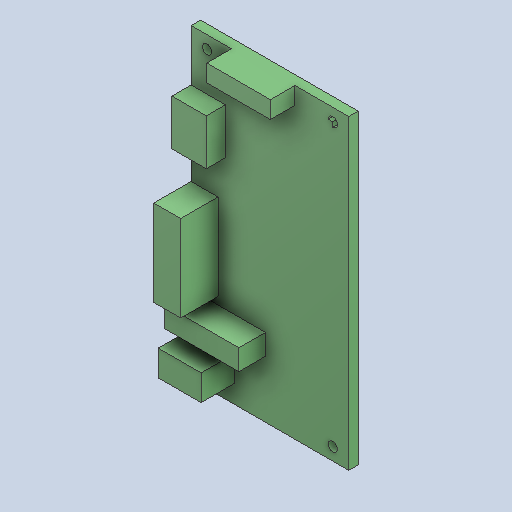
# Autodesk Inventor part: placa
Saved by Autodesk Inventor 2023 (Build 270158000, 158)
## iProperties
Created: 2023-05-12
Part Number: placa
Material: Genérico
Document SubType Name: Modeling
Designer: sergi
Density: 1 g/cm^3
Appearance: Valor por defecto
Author: sergi
Autodesk Inventor part; units mm, degrees
ref_plane "YZ Plane" through (0, 0, 0) normal (1, 0, 0) x (0, 1, 0)
ref_plane "XZ Plane" through (0, 0, 0) normal (0, 1, 0) x (-1, 0, 0)
ref_plane "XY Plane" through (0, 0, 0) normal (0, 0, 1) x (1, 0, 0)
sketch "Boceto1" plane through (0, 0, 0) normal (0, 0, 1) x (1, 0, 0)
  line L0 (27.55, -53.55) -> (-27.55, -53.55)
  line L1 (-27.55, -53.55) -> (-27.55, 53.55)
  line L2 (-27.55, 53.55) -> (27.55, 53.55)
  line L3 (27.55, 53.55) -> (27.55, -53.55)
  line L4 (27.55, -53.55) -> (-27.55, 53.55) construction
  line L5 (-27.55, -53.55) -> (27.55, 53.55) construction
  line L6 (20.325, -47.5) -> (-20.325, -47.5)
  line L7 (-20.325, -47.5) -> (-20.325, 47.5)
  line L8 (-20.325, 47.5) -> (20.325, 47.5)
  line L9 (20.325, 47.5) -> (20.325, -47.5)
  line L10 (20.325, -47.5) -> (-20.325, 47.5) construction
  line L11 (-20.325, -47.5) -> (20.325, 47.5) construction
  line L12 (-20.325, 47.5) -> (-21.975, 47.5)
  line L13 (-21.975, 47.5) -> (-21.975, 49.15)
  line L14 (-21.975, 49.15) -> (-21.975, -49.15)
  line L15 (-21.975, -49.15) -> (21.975, -49.15)
  line L16 (21.975, -49.15) -> (21.975, 49.15)
  line L17 (21.975, 49.15) -> (-21.975, 49.15)
  circle A0 centre (-21.975, 49.15) radius 1.65
  circle A1 centre (21.975, 49.15) radius 1.65
  circle A2 centre (21.975, -49.15) radius 1.65
  circle A3 centre (-21.975, -49.15) radius 1.65
  point P0 (0, 0)
  point P1 (20.325, 49.15)
  point P2 (21.975, 47.5)
  dimension "d0" = 55.1
  dimension "d1" = 107.1
  dimension "d2" = 40.65
  dimension "d3" = 95
  dimension "d4" = 1.65
  dimension "d5" = 1.65
  dimension "d6" = 1.65
  dimension "d7" = 3.3
  dimension "d8" = 3.3
  dimension "d9" = 3.3
  constraints: 36 end point, 6 parallel, 4 coincident, 4 midpoint, 4 perpendicular, 3 centre point, 3 horizontal, 1 vertical alignment, 5 other
  measures "d0" distance of L1.end L2.end
  measures "d1" distance of L0.end L1.end
  measures "d2" distance of L7.end L8.end
  measures "d3" distance of L6.end L7.end
  measures "d4" distance of L7.end L12.end
  measures "d5" distance of L12.end L13.end
  measures "d6" distance between parallel lines of L7 L14
  measures "d7" diameter of A1
  measures "d8" diameter of A2
  measures "d9" diameter of A3
extrude "Extrusión1" add sketch "Boceto1" along normal blind 16.35 contours L0 L1 L2 L3 | A0 L17 A1 L16 A2 L15 A3 L14 | L6 L7 L8 L9 | L17 L16 A1 picked at (20.8888, 49.0276)
sketch "Boceto2" plane through (-27.55, -53.55, 0) normal (-1, 0, 0) x (0, 0, 1)
  line L0 (0, 107.1) -> (0, 88.8)
  line L1 (0, 107.1) -> (0, 0) projected
  line L2 (0, 107.1) -> (3.3, 107.1)
  line L3 (3.3, 107.1) -> (3.3, 53.55)
  line L4 (3.3, 53.55) -> (3.3, 0)
  line L5 (0, 0) -> (16.35, 0) projected
  line L6 (3.3, 107.1) -> (11.9, 107.1)
  line L7 (0, 107.1) -> (16.35, 107.1) projected
  line L8 (11.9, 107.1) -> (11.9, 101.1)
  line L9 (11.9, 101.1) -> (3.3, 101.1)
  line L10 (3.3, 107.1) -> (3.3, 89.1)
  line L11 (0, 102.7) -> (16.35, 102.7) projected
  line L12 (3.3, 107.1) -> (21.3, 107.1) construction
  line L13 (3.3, 89.1) -> (10, 89.1)
  line L14 (10, 89.1) -> (10, 73.1)
  line L15 (10, 73.1) -> (3.3, 73.1)
  line L16 (3.3, 107.1) -> (3.3, 59.9)
  line L17 (3.3, 59.9) -> (16.3, 59.9)
  line L18 (16.3, 59.9) -> (16.35, 59.9)
  line L19 (16.35, 107.1) -> (16.35, 0) projected
  line L20 (16.35, 59.9) -> (16.35, 29.8)
  line L21 (16.35, 59.9) -> (46.45, 59.9) construction
  line L22 (16.35, 29.8) -> (3.3, 29.8)
  line L23 (3.3, 0) -> (3.3, 6.2)
  line L24 (3.3, 6.2) -> (14.8, 6.2)
  line L25 (16.35, 6.05) -> (0, 6.05) projected
  line L26 (3.3, 6.2) -> (14.8, 6.2) construction
  line L27 (14.8, 6.2) -> (14.8, 15.2)
  line L28 (14.8, 6.2) -> (23.8, 6.2) construction
  line L29 (14.8, 15.2) -> (3.3, 15.2)
  line L30 (3.3, 0) -> (3.3, 20)
  line L31 (3.3, 0) -> (23.3, 0) construction
  line L32 (3.3, 20) -> (12.6, 20)
  line L33 (12.6, 20) -> (12.6, 27.2)
  line L34 (12.6, 27.2) -> (3.3, 27.2)
  point P0 (0, 53.55)
  dimension "d17" = 3.3
  dimension "d18" = 8.6
  dimension "d19" = 6
  dimension "d20" = 18
  dimension "d21" = 90
  dimension "d22" = 6.7
  dimension "d23" = 16
  dimension "d24" = 47.2
  dimension "d25" = 13
  dimension "d26" = 90
  dimension "d27" = 30.1
  dimension "d28" = 90
  dimension "d29" = 6.2
  dimension "d30" = 11.5
  dimension "d31" = 0
  dimension "d32" = 9
  dimension "d33" = 90
  dimension "d34" = 20
  dimension "d35" = 90
  dimension "d36" = 9.3
  dimension "d37" = 90
  dimension "d38" = 7.2
  dimension "d39" = 90
  constraints: 58 end point, 13 point on line, 11 perpendicular, 5 equal length, 5 horizontal, 2 collinear, 2 vertical, 1 parallel
  measures "d17" distance of L0.start L2.end
  measures "d18" distance of L2.end L6.end
  measures "d19" distance of L6.end L8.end
  measures "d20" distance of L2.end L10.end
  measures "d21" angle of L10 L12
  measures "d22" distance of L10.end L13.end
  measures "d23" distance of L13.end L14.end
  measures "d24" distance of L2.end L16.end
  measures "d25" distance of L16.end L17.end
  measures "d26" angle of L17 L16
  measures "d27" distance of L18.end L20.end
  measures "d28" angle of L20 L21
  measures "d29" distance of L4.end L23.end
  measures "d30" distance of L23.end L24.end
  measures "d31" distance between parallel lines of L24 L26
  measures "d32" distance of L26.end L27.end
  measures "d33" angle of L28 L27
  measures "d34" distance of L4.end L30.end
  measures "d35" angle of L31 L30
  measures "d36" distance of L30.end L32.end
  measures "d37" angle of L30 L32
  measures "d38" distance of L32.end L33.end
  measures "d39" angle of L33 L32
extrude "Extrusión2" cut sketch "Boceto2" against normal through all contours L7 L19 L11 L8 | L9 L8 L11 L19 L18 L17 L3 L15 L14 L13 | L25 L19 L5 L4 | L4 L24 L27 L29 L32 L33 L34 L22 L19 L25
sketch "Boceto3" plane through (0, 0, 16.35) normal (0, 0, 1) x (1, 0, 0)
  line L0 (-27.55, 53.55) -> (27.55, 53.55) projected
  line L1 (27.55, 47.55) -> (27.55, 35.55) projected
  line L2 (27.55, 53.55) -> (27.55, 47.55) projected
  line L3 (27.55, 35.55) -> (27.55, 19.55) projected
  line L4 (27.55, 19.55) -> (27.55, 6.35) projected
  line L5 (27.55, -23.75) -> (27.55, 6.35) projected
  line L6 (27.55, -26.35) -> (27.55, -33.55) projected
  line L7 (-27.55, 53.55) -> (-27.55, -53.55) projected
  line L8 (27.55, 53.55) -> (-27.55, 53.55) projected
  line L9 (-27.55, -53.55) -> (27.55, -53.55) projected
  line L10 (27.55, -53.55) -> (27.55, 53.55) projected
  line L11 (-27.55, 53.55) -> (-13.45, 53.55)
  line L12 (-21.5719, 47.55) -> (21.975, 47.55) projected
  line L13 (-27.55, 35.55) -> (27.55, 35.55) projected
  line L14 (-27.55, 19.55) -> (27.55, 19.55) projected
  line L15 (-27.55, 6.35) -> (27.55, 6.35) projected
  line L16 (-27.55, -23.75) -> (27.55, -23.75) projected
  line L17 (-27.55, -26.35) -> (27.55, -26.35) projected
  line L18 (-27.55, -33.55) -> (27.55, -33.55) projected
  line L19 (-27.55, -38.35) -> (27.55, -38.35) projected
  line L20 (27.55, -38.35) -> (27.55, -47.35) projected
  line L21 (-27.55, -38.35) -> (27.55, -38.35) projected
  line L22 (-27.55, -47.35) -> (-27.55, -38.35) projected
  line L23 (-27.55, -47.35) -> (27.55, -47.35) projected
  line L24 (27.55, -47.35) -> (27.55, -53.55) projected
  line L25 (-27.55, -47.35) -> (27.55, -47.35) projected
  line L26 (-27.55, -53.55) -> (-27.55, -47.35) projected
  line L27 (27.55, -53.55) -> (-27.55, -53.55) projected
  circle A0 centre (-21.975, -49.15) radius 1.65 projected
  circle A1 centre (21.975, -49.15) radius 1.65 projected
  line L28 (27.55, 53.55) -> (-27.55, 53.55) projected
  line L29 (27.55, 53.55) -> (27.55, 47.55) projected
  line L30 (-27.55, 53.55) -> (27.55, 53.55) projected
  line L31 (-27.55, 47.55) -> (-27.55, 53.55) projected
  line L32 (-27.55, 47.55) -> (-22.3781, 47.55) projected
  arc A2 (-21.5719, 47.55) -> (-22.3781, 47.55) centre (-21.975, 49.15) ccw projected
  line L33 (-21.5719, 47.55) -> (21.975, 47.55) projected
  line L34 (21.975, 49.15) -> (21.975, 47.55) projected
  line L35 (20.325, 49.15) -> (21.975, 49.15) projected
  arc A3 (22.3781, 47.55) -> (20.325, 49.15) centre (21.975, 49.15) ccw projected
  line L36 (22.3781, 47.55) -> (27.55, 47.55) projected
  line L37 (-13.45, 53.55) -> (-13.45, 47.55)
  line L38 (27.55, 53.55) -> (8.75, 53.55)
  line L39 (8.75, 53.55) -> (8.75, 47.55)
  line L40 (-21.5719, 47.55) -> (21.975, 47.55) projected
  line L41 (-27.55, 35.55) -> (-27.55, 47.55) projected
  line L42 (-27.55, 35.55) -> (-15.55, 35.55)
  line L43 (-15.55, 35.55) -> (-15.55, 19.55)
  line L44 (27.55, 6.35) -> (-27.55, 6.35) projected
  line L45 (-27.55, 6.35) -> (-18.15, 6.35)
  line L46 (-18.15, 6.35) -> (-18.15, -26.35)
  line L47 (-27.55, -26.35) -> (-1.55, -26.35)
  line L48 (-1.55, -26.35) -> (-1.55, -33.55)
  line L49 (-27.55, -38.35) -> (-12.55, -38.35)
  line L50 (-12.55, -38.35) -> (-12.55, -47.35)
  point P0 (0, 0)
  point P1 (-18.15, -23.75)
  point P2 (21.975, 47.55)
  dimension "d42" = 14.1
  dimension "d43" = 18.8
  dimension "d44" = 12
  dimension "d45" = 9.4
  dimension "d46" = 26
  dimension "d47" = 15
  constraints: 24 end point, 12 point on line, 6 perpendicular, 2 other
  measures "d42" distance of L0.start L11.end
  measures "d43" distance of L29.start L38.end
  measures "d44" distance of L13.start L42.end
  measures "d45" distance of L15.start L45.end
  measures "d46" distance of L17.start L47.end
  measures "d47" distance of L21.start L49.end
extrude "Extrusión3" cut sketch "Boceto3" against normal up to surface (13.05 mm away) contours L0 L37 L12 A2 L32 L7 | L0 L2 L36 A3 L35 L34 L12 L39 | L13 L3 L14 L43 | L15 L5 L16 L46 | L48 L17 L6 L18 | L19 L10 L23 L50
